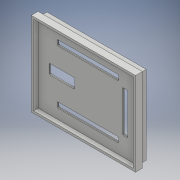
# Autodesk Inventor part: Platform
Saved by Autodesk Inventor 2017 (Build 210142000, 142)
## iProperties
Created: 2018-02-12
Part Number: Platform
Material: Generic
Document SubType Name: Modeling
Designer: Arjuna
Density: 1 g/cm^3
Appearance: Default
Author: Arjuna
Autodesk Inventor part; units mm, degrees
ref_plane "YZ Plane" through (0, 0, 0) normal (1, 0, 0) x (0, 1, 0)
ref_plane "XZ Plane" through (0, 0, 0) normal (0, 1, 0) x (-1, 0, 0)
ref_plane "XY Plane" through (0, 0, 0) normal (0, 0, 1) x (1, 0, 0)
sketch "Sketch1" plane through (0, 0, 0) normal (0, 1, 0) x (-1, 0, 0)
  line L0 (115, 92.5) -> (-115, 92.5)
  line L1 (-115, 92.5) -> (-115, -92.5)
  line L2 (-115, -92.5) -> (115, -92.5)
  line L3 (115, -92.5) -> (115, 92.5)
  point P0 (0, 0)
  dimension "d0" = 230
  dimension "d1" = 185
  dimension "d2" = 92.5
  dimension "d3" = 115
  constraints: 8 end point, 2 parallel, 1 horizontal, 1 perpendicular
  measures "d0" distance of L2.end L1.end
  measures "d1" distance between parallel lines of L2 L0
  measures "d2" distance from line of point (0, 0) L0
  measures "d3" distance from line of point (0, 0) L3
extrude "Extrusion1" add sketch "Sketch1" against normal blind 15
sketch "Sketch5" plane through (0, 0, 0) normal (0, 1, 0) x (1, 0, 0)
  line L0 (-115, -92.5) -> (115, -92.5) projected
  line L1 (115, -92.5) -> (115, 92.5) projected
  line L2 (115, 92.5) -> (-115, 92.5) projected
  line L3 (-115, 92.5) -> (-115, -92.5) projected
  line L4 (-109.5, -87) -> (109.5, -87)
  line L5 (109.5, -87) -> (109.5, 87)
  line L6 (109.5, 87) -> (-109.5, 87)
  line L7 (-109.5, 87) -> (-109.5, -87)
  point P0 (0, 0)
  dimension "d42" = 5.5
  dimension "d43" = 5.5
  dimension "d44" = 5.5
  dimension "d45" = 5.5
  constraints: 8 end point, 2 parallel, 1 horizontal, 1 perpendicular
  measures "d42" distance between parallel lines of L4 L0
  measures "d43" distance between parallel lines of L7 L3
  measures "d44" distance between parallel lines of L2 L6
  measures "d45" distance between parallel lines of L1 L5
extrude "Extrusion6" add sketch "Sketch5" along normal blind 14 contours L7 L6 L5 L4
sketch "Sketch6" plane through (0, 14, 0) normal (0, 1, 0) x (1, 0, 0)
  line L0 (-109.5, -87) -> (109.5, -87) projected
  line L1 (109.5, -87) -> (109.5, 87) projected
  line L2 (109.5, 87) -> (-109.5, 87) projected
  line L3 (-109.5, 87) -> (-109.5, -87) projected
  line L4 (107, -84.5) -> (-107, -84.5)
  line L5 (-107, -84.5) -> (-107, 84.5)
  line L6 (-107, 84.5) -> (107, 84.5)
  line L7 (107, 84.5) -> (107, -84.5)
  point P0 (0, 0)
  dimension "d48" = 2.5
  dimension "d49" = 2.5
  dimension "d50" = 2.5
  dimension "d51" = 2.5
  constraints: 8 end point, 2 parallel, 1 horizontal, 1 perpendicular
  measures "d48" distance between parallel lines of L4 L0
  measures "d49" distance between parallel lines of L3 L5
  measures "d50" distance between parallel lines of L2 L6
  measures "d51" distance between parallel lines of L7 L1
extrude "Extrusion7" cut sketch "Sketch6" against normal blind 15 contours L4 L5 L6 L7
sketch "Sketch7" plane through (0, -15, 0) normal (0, -1, 0) x (1, 0, 0)
  line L0 (115, 92.5) -> (-115, 92.5) projected
  line L1 (-115, 92.5) -> (-115, -92.5) projected
  line L2 (-115, -92.5) -> (115, -92.5) projected
  line L3 (115, -92.5) -> (115, 92.5) projected
  line L4 (110, 87.5) -> (-110, 87.5)
  line L5 (-110, 87.5) -> (-110, -87.5)
  line L6 (-110, -87.5) -> (110, -87.5)
  line L7 (110, -87.5) -> (110, 87.5)
  point P0 (0, 0)
  dimension "d54" = 5
  dimension "d55" = 5
  dimension "d56" = 5
  dimension "d57" = 5
  constraints: 8 end point, 2 parallel, 1 horizontal, 1 perpendicular
  measures "d54" distance between parallel lines of L7 L3
  measures "d55" distance between parallel lines of L2 L6
  measures "d56" distance between parallel lines of L4 L0
  measures "d57" distance between parallel lines of L1 L5
extrude "Extrusion8" cut sketch "Sketch7" against normal blind 10 contours L7 L6 L5 L4
sketch "Sketch8" plane through (0, -1, 0) normal (0, 1, 0) x (1, 0, 0)
  line L0 (107, -84.5) -> (-107, -84.5) projected
  line L1 (107, 84.5) -> (107, -84.5) projected
  line L2 (-107, 84.5) -> (107, 84.5) projected
  line L3 (-107, -84.5) -> (-107, 84.5) projected
  line L4 (-87, -64.5) -> (87, -64.5)
  line L5 (87, -64.5) -> (87, 64.5)
  line L6 (87, 64.5) -> (-87, 64.5)
  line L7 (-87, 64.5) -> (-87, -64.5)
  line L8 (-77, -54.5) -> (77, -54.5)
  line L9 (77, -54.5) -> (77, 54.5)
  line L10 (77, 54.5) -> (-77, 54.5)
  line L11 (-77, 54.5) -> (-77, -54.5)
  line L12 (-87, -44.5) -> (-77, -44.5)
  line L13 (-67, -64.5) -> (-67, -54.5)
  line L14 (-87, 44.5) -> (-77, 44.5)
  line L15 (-67, 54.5) -> (-67, 64.5)
  line L16 (67, -64.5) -> (67, -54.5)
  line L17 (77, -44.5) -> (87, -44.5)
  line L18 (67, 54.5) -> (67, 64.5)
  line L19 (77, 44.5) -> (87, 44.5)
  point P0 (0, 0)
  dimension "d60" = 20
  dimension "d61" = 20
  dimension "d62" = 20
  dimension "d63" = 20
  dimension "d64" = 10
  dimension "d65" = 10
  dimension "d66" = 10
  dimension "d67" = 10
  dimension "d68" = 20
  dimension "d69" = 20
  dimension "d70" = 20
  dimension "d71" = 20
  dimension "d72" = 20
  dimension "d73" = 20
  dimension "d74" = 20
  dimension "d75" = 20
  constraints: 32 end point, 16 point on line, 10 perpendicular, 4 parallel, 2 horizontal
  measures "d60" distance between parallel lines of L4 L0
  measures "d61" distance between parallel lines of L2 L6
  measures "d62" distance between parallel lines of L7 L3
  measures "d63" distance between parallel lines of L1 L5
  measures "d64" distance between parallel lines of L8 L4
  measures "d65" distance between parallel lines of L11 L7
  measures "d66" distance between parallel lines of L6 L10
  measures "d67" distance between parallel lines of L5 L9
  measures "d68" distance between parallel lines of L12 L4
  measures "d69" distance between parallel lines of L13 L7
  measures "d70" distance between parallel lines of L6 L14
  measures "d71" distance between parallel lines of L15 L7
  measures "d72" distance between parallel lines of L5 L16
  measures "d73" distance between parallel lines of L17 L4
  measures "d74" distance between parallel lines of L5 L18
  measures "d75" distance between parallel lines of L6 L19
extrude "Extrusion9" cut sketch "Sketch8" against normal through all contours L13 L8 L16 L4 | L17 L9 L19 L5 | L6 L18 L10 L15
sketch "Sketch9" plane through (0, -1, 0) normal (0, 1, 0) x (1, 0, 0)
  line L0 (67, -54.5) -> (67, -64.5) projected
  line L1 (67, -64.5) -> (-67, -64.5) projected
  line L2 (-67, -64.5) -> (-67, -54.5) projected
  line L3 (-67, -54.5) -> (67, -54.5) projected
  line L4 (87, 44.5) -> (87, -44.5) projected
  line L5 (87, -44.5) -> (77, -44.5) projected
  line L6 (77, -44.5) -> (77, 44.5) projected
  line L7 (77, 44.5) -> (87, 44.5) projected
  line L8 (67, 64.5) -> (67, 54.5) projected
  line L9 (67, 54.5) -> (-67, 54.5) projected
  line L10 (-67, 54.5) -> (-67, 64.5) projected
  line L11 (-67, 64.5) -> (67, 64.5) projected
  line L12 (107, -84.5) -> (-107, -84.5) projected
  line L13 (107, 84.5) -> (107, -84.5) projected
  line L14 (-107, 84.5) -> (107, 84.5) projected
  line L15 (-107, -84.5) -> (-107, 84.5) projected
  line L16 (-85, -10) -> (-30, -10)
  line L17 (-30, -10) -> (-30, 10)
  line L18 (-30, 10) -> (-85, 10)
  line L19 (-85, 10) -> (-85, -10)
  point P0 (0, 0)
  dimension "d78" = 55
  dimension "d79" = 20
  dimension "d80" = 30
  dimension "d81" = 10
  constraints: 8 end point, 2 parallel, 1 horizontal, 1 perpendicular
  measures "d78" distance of L18.end L17.end
  measures "d79" distance between parallel lines of L18 L16
  measures "d80" distance from line of point (0, 0) L17
  measures "d81" distance from line of point (0, 0) L16
extrude "Extrusion10" cut sketch "Sketch9" against normal through all contours L19 L18 L17 L16
fillet "Fillet1" radius 1 48 edges at (-57.5, -1, -10) (-57.5, -1, 10) (-85, -1, 0) (-30, -1, 0) (0, -1, 54.5) (0, -1, -54.5) (77, -1, 0) (77, -5, 0) (0, -5, 54.5) (0, -5, -54.5) (-85, -5, 0) (-57.5, -5, -10) (-57.5, -5, 10) (-30, -5, 0) (-85, -3, -10) (-85, -3, 10) (-30, -3, 10) (-30, -3, -10) (-67, -3, 54.5) (67, -3, 54.5) (77, -3, 44.5) (77, -3, -44.5) (67, -3, -54.5) (-67, -3, -54.5) (-67, -5, 59.5) (0, -5, 64.5) (67, -5, 59.5) (-67, -5, -59.5) (0, -5, -64.5) (67, -5, -59.5) (82, -5, -44.5) (87, -5, 0) (82, -5, 44.5) (-67, -1, 59.5) (0, -1, 64.5) (67, -1, 59.5) (-67, -1, -59.5) (0, -1, -64.5) (67, -1, -59.5) (82, -1, 44.5) (87, -1, 0) (82, -1, -44.5) (87, -3, -44.5) (87, -3, 44.5) (67, -3, 64.5) (-67, -3, 64.5) (-67, -3, -64.5) (67, -3, -64.5)
equation "\"d2\" = 0.5 * d1"
equation "\"d3\" = 0.5 * d0"
equation "\"d43\" = d42"
equation "\"d44\" = d42"
equation "\"d45\" = d42"
equation "\"d49\" = d48"
equation "\"d50\" = d48"
equation "\"d51\" = d48"
equation "\"d55\" = d54"
equation "\"d56\" = d54"
equation "\"d57\" = d54"
equation "\"d61\" = d60"
equation "\"d62\" = d60"
equation "\"d63\" = d60"
equation "\"d65\" = d64"
equation "\"d66\" = d64"
equation "\"d67\" = d64"
equation "\"d68\" = d69"
equation "\"d70\" = d69"
equation "\"d71\" = d69"
equation "\"d72\" = d69"
equation "\"d73\" = d69"
equation "\"d74\" = d69"
equation "\"d75\" = d69"
equation "\"d81\" = 0.5 * d79"
body "Solid1"
